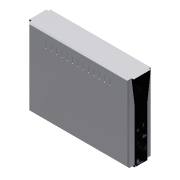
# Autodesk Inventor part: Wireless Router
Saved by Autodesk Inventor 2015 (Build 190159000, 159)
## iProperties
Created: 2015-01-11
Part Number: Wireless Router
Material: Generic
Document SubType Name: Modeling
Designer: Peter
Density: 1 g/cm^3
Appearance: Snow
Author: Peter
Autodesk Inventor part; units mm, degrees
ref_plane "YZ Plane" through (0, 0, 0) normal (1, 0, 0) x (0, 1, 0)
ref_plane "XZ Plane" through (0, 0, 0) normal (0, 1, 0) x (-1, 0, 0)
ref_plane "XY Plane" through (0, 0, 0) normal (0, 0, 1) x (1, 0, 0)
sketch "Sketch1" plane through (0, 0, 0) normal (0, 0, 1) x (1, 0, 0)
  line L0 (0, 0) -> (119.38, 0)
  line L1 (119.38, 0) -> (119.38, 91.44)
  line L2 (119.38, 91.44) -> (0, 91.44)
  line L3 (0, 91.44) -> (0, 0)
  dimension "d0" = 119.38
  dimension "d1" = 91.44
  constraints: 8 end point, 2 parallel, 1 horizontal, 1 perpendicular
  measures "d0" distance of L1.end L2.end
  measures "d1" distance of L0.end L1.end
extrude "Extrusion1" add sketch "Sketch1" along normal blind 27.94
chamfer "Chamfer1" distance 1.27 angle 45 1 edges at (59.69, 0, 0)
chamfer "Chamfer2" distance 1.27 angle 45 1 edges at (0, 46.355, 0)
chamfer "Chamfer3" distance 1.27 angle 45 1 edges at (60.325, 91.44, 0)
chamfer "Chamfer4" distance 1.27 angle 45 1 edges at (119.38, 45.72, 0)
chamfer "Chamfer5" distance 1.27 angle 45 1 edges at (0, 45.72, 27.94)
chamfer "Chamfer6" distance 1.27 angle 45 1 edges at (60.325, 0, 27.94)
chamfer "Chamfer7" distance 1.27 angle 45 2 edges at (60.325, 91.44, 27.94) (119.38, 46.355, 27.94)
sketch "Sketch2" plane through (119.38, 0, 1.27) normal (1, 0, 0) x (0, 0, -1)
  line L0 (-25.4, 0) -> (-25.4, 91.44) projected
  line L1 (0, 0) -> (-25.4, 0) projected
  line L2 (-19.05, 0) -> (-19.05, 60.96)
  line L3 (-6.35, 0) -> (-6.35, 60.96)
  line L4 (-19.05, 0) -> (-6.35, 0)
  line L5 (-19.05, 60.96) -> (-22.86, 91.44)
  line L6 (0, 91.44) -> (-25.4, 91.44) projected
  line L7 (-6.35, 60.96) -> (-2.54, 91.44)
  line L8 (-22.86, 91.44) -> (-2.54, 91.44)
  dimension "d25" = 60.96
  dimension "d26" = 60.96
  dimension "d27" = 12.7
  dimension "d28" = 6.35
  dimension "d29" = 20.32
  dimension "d30" = 2.54
  constraints: 12 end point, 4 point on line, 2 vertical, 1 collinear, 1 horizontal
  measures "d25" distance of L2.start L2.end
  measures "d26" distance of L3.start L3.end
  measures "d27" distance of L3.start L2.start
  measures "d28" distance between parallel lines of L2 L0
  measures "d29" distance of L7.end L5.end
  measures "d30" distance of L0.end L5.end
extrude "Extrusion2" add sketch "Sketch2" along normal blind 2.54 contours L2 L5 L6 L7 L3 L1
sketch "Sketch3" plane through (0, 0, 1.27) normal (0, -1, 0) x (1, 0, 0)
  line L0 (0, 0) -> (0, 25.4) projected
  line L1 (119.38, 19.05) -> (0, 19.05)
  line L2 (119.38, 6.35) -> (0, 6.35)
  line L3 (0, 19.05) -> (0, 6.35)
  line L4 (119.38, 19.05) -> (119.38, 6.35)
  constraints: 8 end point, 2 perpendicular, 2 point on line, 1 collinear, 1 vertical
extrude "Extrusion3" add sketch "Sketch3" along normal blind 2.54
sketch "Sketch4" plane through (0, 0, 1.27) normal (-1, 0, 0) x (0, 0, 1)
  line L0 (25.4, 91.44) -> (25.4, 0) projected
  line L1 (0, 91.44) -> (25.4, 91.44) projected
  line L2 (0, 0) -> (0, 91.44) projected
  line L3 (0, 0) -> (6.35, 0) projected
  line L4 (6.35, 0) -> (6.35, -2.54) projected
  line L5 (19.05, -2.54) -> (6.35, -2.54) projected
  line L6 (19.05, 0) -> (19.05, -2.54) projected
  line L7 (19.05, 0) -> (25.4, 0) projected
sketch "Sketch5" plane through (121.92, 0, 1.27) normal (1, 0, 0) x (0, 0, -1)
  line L0 (-2.54, 91.44) -> (-22.86, 91.44) projected
  line L1 (-22.86, 91.44) -> (-19.05, 60.96) projected
  line L2 (-19.05, 60.96) -> (-19.05, 0) projected
  line L3 (-19.05, 0) -> (-6.35, 0) projected
  line L4 (-6.35, 0) -> (-6.35, 60.96) projected
  line L5 (-6.35, 60.96) -> (-2.54, 91.44) projected
sketch "Sketch6" plane through (0, 0, 1.27) normal (-1, 0, 0) x (0, 0, 1)
  line L0 (25.4, 91.44) -> (25.4, 0) projected
  line L1 (0, 91.44) -> (25.4, 91.44) projected
  line L2 (19.05, -2.54) -> (6.35, -2.54) projected
  line L3 (6.35, 0) -> (6.35, 60.96)
  line L4 (6.35, 0) -> (6.35, 60.96) projected
  line L5 (19.05, 60.96) -> (19.05, 0)
  line L6 (19.05, 0) -> (6.35, 0)
  line L7 (6.35, 60.96) -> (2.54, 91.44)
  line L8 (2.54, 91.44) -> (6.35, 60.96) projected
  line L9 (19.05, 60.96) -> (22.86, 91.44)
  line L10 (2.54, 91.44) -> (22.86, 91.44)
  dimension "d35" = 60.96
  dimension "d36" = 2.54
  dimension "d37" = 6.35
  constraints: 12 end point, 3 equal length, 1 horizontal, 1 point on line
  measures "d35" distance of L5.start L5.end
  measures "d36" distance of L0.start L9.end
  measures "d37" distance from line of L0 L5.start
extrude "Extrusion4" add sketch "Sketch6" along normal blind 2.54
sketch "Sketch7" plane through (0, 0, 27.94) normal (0, 0, 1) x (1, 0, 0)
  line L0 (1.27, 90.17) -> (118.11, 90.17) projected
  line L1 (20.32, 82.55) -> (20.32, 74.93)
  line L2 (20.32, 74.93) -> (21.59, 74.93)
  line L3 (21.59, 74.93) -> (21.59, 82.55)
  line L4 (21.59, 82.55) -> (20.32, 82.55)
  line L5 (0, 91.44) -> (0, 0) projected
  line L6 (26.67, 82.55) -> (26.67, 74.93)
  line L7 (26.67, 74.93) -> (27.94, 74.93)
  line L8 (27.94, 74.93) -> (27.94, 82.55)
  line L9 (27.94, 82.55) -> (26.67, 82.55)
  line L10 (33.02, 82.55) -> (33.02, 74.93)
  line L11 (33.02, 74.93) -> (34.29, 74.93)
  line L12 (34.29, 74.93) -> (34.29, 82.55)
  line L13 (34.29, 82.55) -> (33.02, 82.55)
  line L14 (39.37, 82.55) -> (39.37, 74.93)
  line L15 (39.37, 74.93) -> (40.64, 74.93)
  line L16 (40.64, 74.93) -> (40.64, 82.55)
  line L17 (40.64, 82.55) -> (39.37, 82.55)
  line L18 (45.72, 82.55) -> (45.72, 74.93)
  line L19 (45.72, 74.93) -> (46.99, 74.93)
  line L20 (46.99, 74.93) -> (46.99, 82.55)
  line L21 (46.99, 82.55) -> (45.72, 82.55)
  line L22 (52.07, 82.55) -> (52.07, 74.93)
  line L23 (52.07, 74.93) -> (53.34, 74.93)
  line L24 (53.34, 74.93) -> (53.34, 82.55)
  line L25 (53.34, 82.55) -> (52.07, 82.55)
  line L26 (58.42, 82.55) -> (58.42, 74.93)
  line L27 (58.42, 74.93) -> (59.69, 74.93)
  line L28 (59.69, 74.93) -> (59.69, 82.55)
  line L29 (59.69, 82.55) -> (58.42, 82.55)
  line L30 (64.77, 82.55) -> (64.77, 74.93)
  line L31 (64.77, 74.93) -> (66.04, 74.93)
  line L32 (66.04, 74.93) -> (66.04, 82.55)
  line L33 (66.04, 82.55) -> (64.77, 82.55)
  line L34 (71.12, 82.55) -> (71.12, 74.93)
  line L35 (71.12, 74.93) -> (72.39, 74.93)
  line L36 (72.39, 74.93) -> (72.39, 82.55)
  line L37 (72.39, 82.55) -> (71.12, 82.55)
  line L38 (77.47, 82.55) -> (77.47, 74.93)
  line L39 (77.47, 74.93) -> (78.74, 74.93)
  line L40 (78.74, 74.93) -> (78.74, 82.55)
  line L41 (78.74, 82.55) -> (77.47, 82.55)
  line L42 (83.82, 82.55) -> (83.82, 74.93)
  line L43 (83.82, 74.93) -> (85.09, 74.93)
  line L44 (85.09, 74.93) -> (85.09, 82.55)
  line L45 (85.09, 82.55) -> (83.82, 82.55)
  line L46 (90.17, 82.55) -> (90.17, 74.93)
  line L47 (90.17, 74.93) -> (91.44, 74.93)
  line L48 (91.44, 74.93) -> (91.44, 82.55)
  line L49 (91.44, 82.55) -> (90.17, 82.55)
  line L50 (96.52, 82.55) -> (96.52, 74.93)
  line L51 (96.52, 74.93) -> (97.79, 74.93)
  line L52 (97.79, 74.93) -> (97.79, 82.55)
  line L53 (97.79, 82.55) -> (96.52, 82.55)
  dimension "d40" = 7.62
  dimension "d41" = 1.27
  dimension "d42" = 7.62
  dimension "d44" = 20.32
  dimension "d47" = 6.35
  constraints: 104 end point, 2 horizontal, 2 perpendicular, 1 vertical, 96 other
  measures "d40" distance of L1.start L1.end
  measures "d41" distance of L1.end L2.end
  measures "d42" distance from line of L0 L1.start
  measures "d44" distance from line of L5 L1.start
  measures "d47" distance of L3.end L9.start
extrude "Extrusion5" cut sketch "Sketch7" against normal blind 3.175
body "Solid1"
